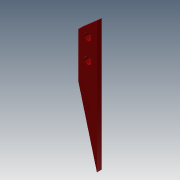
# Autodesk Inventor part: packa
Saved by Autodesk Inventor 2013 (Build 170138000, 138)
## iProperties
Created: 2013-02-02
Part Number: packa
Material: Generic
Document SubType Name: Modeling
Designer: idle-rug
Density: 1 g/cm^3
Author: idle-rug
Autodesk Inventor part; units mm, degrees
ref_plane "YZ Plane" through (0, 0, 0) normal (1, 0, 0) x (0, 1, 0)
ref_plane "XZ Plane" through (0, 0, 0) normal (0, 1, 0) x (-1, 0, 0)
ref_plane "XY Plane" through (0, 0, 0) normal (0, 0, 1) x (1, 0, 0)
sketch "Sketch1" plane through (0, 0, 0) normal (0, 1, 0) x (-1, 0, 0)
  line L0 (-4, 15) -> (4, 15)
  line L1 (-4, -15) -> (-4, 15)
  line L2 (4, 15) -> (-4, -15) construction
  line L3 (-4, -15) -> (4, 15)
  line L4 (-4, 15) -> (-4, 42)
  line L5 (0, 15) -> (0, 25)
  circle A0 centre (0, 25) radius 1.5
  line L6 (4, 15) -> (4, 35)
  line L7 (4, 35) -> (-4, 42)
  line L8 (0, 25) -> (0, 34)
  circle A1 centre (0, 34) radius 1.5
  point P0 (0, 0)
  dimension "d2" = 27
  dimension "d9" = 10
  dimension "d10" = 3
  dimension "d13" = 20
  dimension "d14" = 9
  dimension "d15" = 3
  constraints: 18 end point, 2 centre point, 2 coincident, 2 collinear, 2 midpoint, 1 horizontal, 1 parallel
  measures "d2" distance of L0.start L4.end
  measures "d9" distance of L5.start L5.end
  measures "d10" diameter of A0
  measures "d13" distance of L0.end L6.end
  measures "d14" distance of L8.start L8.end
  measures "d15" diameter of A1
extrude "Extrusion1" add sketch "Sketch1" along normal blind 2
body "Solid1"
